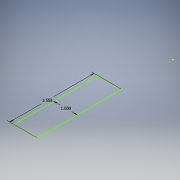
# Autodesk Inventor part: Part16
Saved by Autodesk Inventor 2018 (Build 220112000, 112)
## iProperties
Created: 2018-05-09
Part Number: Part16
Material: Generic
Document SubType Name: Modeling
Designer: Administrator
Density: 1 g/cm^3
Appearance: Default
Author: Administrator
Autodesk Inventor part; units mm, degrees
ref_plane "YZ Plane" through (0, 0, 0) normal (1, 0, 0) x (0, 1, 0)
ref_plane "XZ Plane" through (0, 0, 0) normal (0, 1, 0) x (-1, 0, 0)
ref_plane "XY Plane" through (0, 0, 0) normal (0, 0, 1) x (1, 0, 0)
sketch "Sketch1" plane through (0, 0, 0) normal (0, 1, 0) x (-1, 0, 0)
  line L0 (25.8542, 137.6723) -> (0.4542, 137.6723)
  line L1 (0.4542, 137.6723) -> (0.4542, 55.1223)
  line L2 (0.4542, 55.1223) -> (25.8542, 55.1223)
  line L3 (25.8542, 55.1223) -> (25.8542, 137.6723)
  line L4 (25.8542, 137.6723) -> (30.6167, 137.6723)
  line L5 (30.6167, 137.6723) -> (30.6167, 132.9098)
  line L6 (30.6167, 132.9098) -> (25.8542, 132.9098)
  line L7 (25.8542, 132.9098) -> (25.8542, 137.6723)
  line L8 (25.8542, 118.2254) -> (30.1625, 118.2254)
  line L9 (30.1625, 118.2254) -> (30.1625, 113.4629)
  line L10 (30.1625, 113.4629) -> (25.8542, 113.4629)
  line L11 (25.8542, 113.4629) -> (25.8542, 118.2254)
  line L12 (25.8542, 98.7785) -> (30.6167, 98.7785)
  line L13 (30.6167, 98.7785) -> (30.6167, 94.016)
  line L14 (30.6167, 94.016) -> (25.8542, 94.016)
  line L15 (25.8542, 94.016) -> (25.8542, 98.7785)
  line L16 (25.8542, 55.1223) -> (30.6167, 55.1223)
  line L17 (30.6167, 55.1223) -> (30.6167, 59.8848)
  line L18 (30.6167, 59.8848) -> (25.8542, 59.8848)
  line L19 (25.8542, 59.8848) -> (25.8542, 55.1223)
  line L20 (25.8542, 79.3316) -> (30.1625, 79.3316)
  line L21 (30.1625, 79.3316) -> (30.1625, 74.5691)
  line L22 (30.1625, 74.5691) -> (25.8542, 74.5691)
  line L23 (25.8542, 74.5691) -> (25.8542, 79.3316)
  line L24 (0.4542, 137.6723) -> (-4.3083, 137.6723)
  line L25 (-4.3083, 137.6723) -> (-4.3083, 132.9098)
  line L26 (-4.3083, 132.9098) -> (0.4542, 132.9098)
  line L27 (0.4542, 132.9098) -> (0.4542, 137.6723)
  line L28 (0.4542, 118.2254) -> (-4.3083, 118.2254)
  line L29 (-4.3083, 118.2254) -> (-4.3083, 113.4629)
  line L30 (-4.3083, 113.4629) -> (0.4542, 113.4629)
  line L31 (0.4542, 113.4629) -> (0.4542, 118.2254)
  line L32 (0.4542, 98.7785) -> (-4.3083, 98.7785)
  line L33 (-4.3083, 98.7785) -> (-4.3083, 94.016)
  line L34 (-4.3083, 94.016) -> (0.4542, 94.016)
  line L35 (0.4542, 94.016) -> (0.4542, 98.7785)
  line L36 (0.4542, 79.3316) -> (-4.3083, 79.3316)
  line L37 (-4.3083, 79.3316) -> (-4.3083, 74.5691)
  line L38 (-4.3083, 74.5691) -> (0.4542, 74.5691)
  line L39 (0.4542, 74.5691) -> (0.4542, 79.3316)
  line L40 (0.4542, 59.8848) -> (-4.3083, 59.8848)
  line L41 (-4.3083, 59.8848) -> (-4.3083, 55.1223)
  line L42 (-4.3083, 55.1223) -> (0.4542, 55.1223)
  line L43 (0.4542, 55.1223) -> (0.4542, 59.8848)
  point P0 (0, 0)
  dimension "d0" = 82.55
  dimension "d1" = 25.4
  dimension "d2" = 4.7625
  dimension "d3" = 4.7625
  dimension "d4" = 4.7625
  dimension "d5" = 14.6844
  dimension "d6" = 4.7625
  dimension "d7" = 4.7625
  dimension "d8" = 14.6844
  dimension "d9" = 14.6844
  dimension "d10" = 4.7625
  dimension "d11" = 4.7625
  constraints: 88 end point, 22 parallel, 11 horizontal, 11 perpendicular, 11 point on line
  measures "d0" distance of L0.end L1.end
  measures "d1" distance between parallel lines of L1 L3
  measures "d2" distance between parallel lines of L3 L5
  measures "d3" distance between parallel lines of L4 L6
  measures "d4" distance between parallel lines of L10 L8
  measures "d5" distance between parallel lines of L6 L8
  measures "d6" distance between parallel lines of L18 L16
  measures "d7" distance between parallel lines of L14 L12
  measures "d8" distance between parallel lines of L10 L12
  measures "d9" distance between parallel lines of L14 L20
  measures "d10" distance between parallel lines of L22 L20
  measures "d11" distance between parallel lines of L1 L25
extrude "Extrusion1" add sketch "Sketch1" along normal blind 4.7625
body "Solid1"
